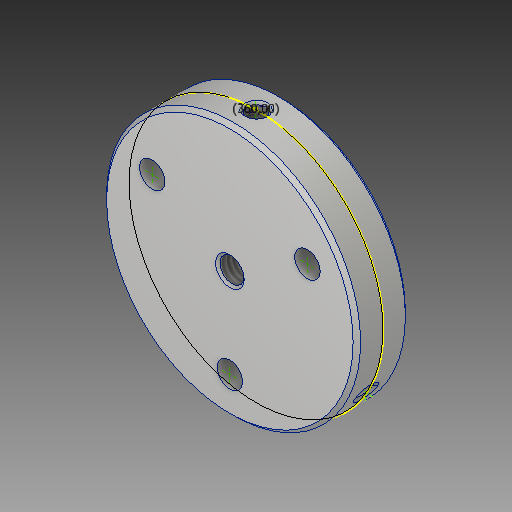
# Autodesk Inventor part: srodek_pajaka
Saved by Autodesk Inventor 2019.4 (Build 234330000, 330)
## iProperties
Created: 2019-05-25
Part Number: srodek_pajaka
Material: Aluminum 6061
Document SubType Name: Modeling
Designer: Esterka
Density: 2.7 g/cm^3
Appearance: Aluminum - Flat
Author: Esterka
Autodesk Inventor part; units mm, degrees
ref_plane "YZ Plane" through (0, 0, 0) normal (1, 0, 0) x (0, 1, 0)
ref_plane "XY Plane" through (0, 0, 0) normal (0, 0, 1) x (1, 0, 0)
sketch "Sketch2" plane through (0, 0, 0) normal (0, 0, 1) x (1, 0, 0)
  circle A0 centre (0, 0) radius 17
  dimension "d0" = 34
  constraints: 1 centre point, 1 coincident
  measures "d0" diameter of A0
extrude "Extrusion1" add sketch "Sketch2" along normal mid plane 7
ref_plane "Work Plane2" through (0, 17, 0) normal (0, 1, 0) x (-1, 0, 0)
sketch "Sketch3" plane through (0, 17, 0) normal (0, 1, 0) x (-1, 0, 0)
  point P0 (0, 0)
  point P1 (0, 0)
  constraints: 1 coincident
sketch "Sketch4" plane through (0, 0, 0) normal (0, 0, 1) x (1, 0, 0)
  circle A0 centre (0, 0) radius 17 projected
  point P0 (0, 17)
  point P1 (0, 17)
  point P2 (0, 17)
  point P3 (-14.7224, -8.5)
  point P4 (-14.7224, -8.5)
  point P5 (-14.7224, -8.5)
  point P6 (14.7224, -8.5)
  point P7 (14.7224, -8.5)
  point P8 (14.7224, -8.5)
  dimension "d5" = 360
  constraints: 6 coincident, 1 vertical alignment, 11 other
ref_plane "Work Plane3" through (14.7224, -8.5, 0) normal (0.8660254, -0.5, 0) x (0.5, 0.8660254, 0)
ref_plane "Work Plane4" through (-14.7224, -8.5, 0) normal (-0.8660254, -0.5, 0) x (0.5, -0.8660254, 0)
sketch "Sketch5" plane through (-14.7224, -8.5, 0) normal (-0.8660254, -0.5, 0) x (0.5, -0.8660254, 0)
  point P0 (0, 0)
ref_plane "Work Plane5" through (0, 0, 0) normal (0, 0, 1) x (1, 0, 0)
sketch "Sketch8" plane through (0, 0, 3.5) normal (0, 0, 1) x (1, 0, 0)
  circle A0 centre (0, 0) radius 12
  point P0 (0, -12)
  point P1 (10.3923, 6)
  point P2 (-10.3923, 6)
  dimension "d7" = 24
  dimension "d10" = 360
  constraints: 1 coincident, 1 vertical alignment, 6 other
sketch "Sketch9" plane through (0, 0, 0) normal (0, 0, 1) x (1, 0, 0)
  point P0 (0, 0)
hole "Hole3" at (0, 0, 3.5) direction (0, 0, -1) diameter 3.242 end through all start extended yes thread size "M4x0.7" class "6H" standard "ISO Metric profile"
sketch "Sketch12" plane through (0, 17, 0) normal (0, 1, 0) x (-1, 0, 0)
  point P0 (0, 0)
sketch "Sketch13" plane through (0, 17, 0) normal (0, 1, 0) x (-1, 0, 0)
  point P0 (0, 0)
  point P1 (0, 0)
  constraints: 1 coincident
hole "Hole4" at (0, 17, 0) direction (0, -1, 0) diameter 2.459 depth 8.8 tip angle 118 thread size "M3x0.5" class "6H" standard "ISO Metric profile"
pattern_circular "Circular Pattern1" count 3 over 360 about axis through (0, 0, -10) along (0, 0, 1) of "Hole4"
chamfer "Chamfer1" distance 0.3 angle 45 10 edges at (0, 1.621, -3.5) (0, 1.621, 3.5) (0.922, 16.975, 0.8134) (0.9217, 16.975, -0.8138) (-0.9219, 16.975, 0.8135) (-0.9221, 16.975, -0.8133) (15.2986, -7.413, -0.0002) (14.0691, -9.5425, 0.002) (-14.0691, -9.5425, -0.0002) (-15.2986, -7.413, 0.002)
chamfer "Chamfer2" distance 0.5 angle 45 2 edges at (-17, 0, 3.5) (-17, 0, -3.5)
sketch "Sketch14" plane through (0, 0, -3.5) normal (0, 0, -1) x (-1, 0, 0)
  point P0 (0, 0)
  point P1 (0, -12)
  point P2 (10.3923, 6)
  point P3 (-10.3923, 6)
  dimension "d42" = 12
  dimension "d45" = 360
  constraints: 4 other
  measures "d42" distance of point (0, 0) point (0, -12)
hole "Hole5" at (-10.3923, 6, -3.5) at (10.3923, 6, -3.5) at (0, -12, -3.5) direction (0, 0, 1) diameter 3.4 end through all countersink diameter 6.3 countersink angle 90 clearance for "Countersunk Flat Head Screw ISO 2009/7046" size "M3" standard "ISO"
sketch "Sketch10" plane through (0, 0, 3.5) normal (0, 0, 1) x (1, 0, 0)
  point P0 (10.3923, 6)
  point P1 (0, -12)
  point P2 (-10.3923, 6)
body "Solid1"
